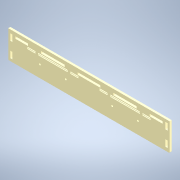
# Autodesk Inventor part: case bottom front
Saved by Autodesk Inventor 2022 (Build 260153000, 153)
## iProperties
Created: 2021-05-28
Part Number: case bottom front
Material: Nylon, molybdenum disulphide
Document SubType Name: Modeling
Designer: benka
Density: 1.13 g/cm^3
Appearance: Nylon 6
Author: benka
Autodesk Inventor part; units mm, degrees
ref_plane "YZ Plane" through (0, 0, 0) normal (1, 0, 0) x (0, 1, 0)
ref_plane "XZ Plane" through (0, 0, 0) normal (0, 1, 0) x (-1, 0, 0)
ref_plane "XY Plane" through (0, 0, 0) normal (0, 0, 1) x (1, 0, 0)
sketch "Sketch1" plane through (0, 0, 0) normal (0, 0, 1) x (1, 0, 0)
  circle A0 centre (-5.8379, -1.3582) radius 2
  circle A1 centre (54.1621, -1.3582) radius 2
  line L0 (81.6621, 21.6418) -> (111.6621, 21.6418) projected
  line L1 (111.6621, 21.6418) -> (111.6621, 26.6418) projected
  line L2 (81.6621, 26.6418) -> (111.6621, 26.6418) projected
  line L3 (81.6621, 21.6418) -> (81.6621, 26.6418) projected
  line L4 (-3.3379, 21.6418) -> (51.6621, 21.6418) projected
  line L5 (51.6621, 21.6418) -> (51.6621, 26.6418) projected
  line L6 (-3.3379, 26.6418) -> (51.6621, 26.6418) projected
  line L7 (-3.3379, 21.6418) -> (-3.3379, 26.6418) projected
  line L8 (-86.3379, 21.6418) -> (-33.3379, 21.6418) projected
  line L9 (-33.3379, 21.6418) -> (-33.3379, 26.6418) projected
  line L10 (-86.3379, 26.6418) -> (-33.3379, 26.6418) projected
  line L11 (-86.3379, 21.6418) -> (-86.3379, 26.6418) projected
  line L12 (-171.3379, 21.6418) -> (-116.3379, 21.6418) projected
  line L13 (-116.3379, 21.6418) -> (-116.3379, 26.6418) projected
  line L14 (-171.3379, 26.6418) -> (-116.3379, 26.6418) projected
  line L15 (-171.3379, 21.6418) -> (-171.3379, 26.6418) projected
  line L16 (-231.3379, 21.6418) -> (-201.3379, 21.6418) projected
  line L17 (-201.3379, 21.6418) -> (-201.3379, 26.6418) projected
  line L18 (-231.3379, 26.6418) -> (-201.3379, 26.6418) projected
  line L19 (-231.3379, 21.6418) -> (-231.3379, 26.6418) projected
  line L20 (126.1621, -31.3589) -> (-245.8379, -31.3589)
  line L21 (-247.8379, -29.3589) -> (-247.8379, 34.6418)
  line L22 (128.1621, -29.3589) -> (128.1621, 34.6418)
  line L23 (-247.8379, 34.6418) -> (128.1621, 34.6418)
  arc A2 (-247.8379, -29.3589) -> (-245.8379, -31.3589) centre (-245.8379, -29.3589) ccw
  arc A3 (126.1621, -31.3589) -> (128.1621, -29.3589) centre (126.1621, -29.3589) ccw
  line L24 (123.1621, -23.3589) -> (123.1621, -8.3597) projected
  line L25 (123.1621, -8.3597) -> (118.1621, -8.3597) projected
  line L26 (118.1621, -23.3589) -> (118.1621, -8.3597) projected
  line L27 (123.1621, -23.3589) -> (118.1621, -23.3589) projected
  line L28 (123.1621, 11.6403) -> (123.1621, 26.6418) projected
  line L29 (123.1621, 26.6418) -> (118.1621, 26.6418) projected
  line L30 (118.1621, 11.6403) -> (118.1621, 26.6418) projected
  line L31 (123.1621, 11.6403) -> (118.1621, 11.6403) projected
  line L32 (-237.8379, -23.3589) -> (-237.8379, -8.3597) projected
  line L33 (-237.8379, -8.3597) -> (-242.8379, -8.3597) projected
  line L34 (-242.8379, -23.3589) -> (-242.8379, -8.3597) projected
  line L35 (-237.8379, -23.3589) -> (-242.8379, -23.3589) projected
  line L36 (-237.8379, 11.6403) -> (-237.8379, 26.6418) projected
  line L37 (-237.8379, 26.6418) -> (-242.8379, 26.6418) projected
  line L38 (-242.8379, 11.6403) -> (-242.8379, 26.6418) projected
  line L39 (-237.8379, 11.6403) -> (-242.8379, 11.6403) projected
  line L40 (-201.8409, 14.8575) -> (-185.8409, 14.8575)
  line L41 (-185.8409, 19.8575) -> (-201.8409, 19.8575)
  line L42 (-85.8409, 14.8575) -> (-101.8409, 14.8575)
  line L43 (-101.8409, 19.8575) -> (-85.8409, 19.8575)
  line L44 (-176.8409, 14.8575) -> (-110.8409, 14.8575)
  line L45 (-110.8409, 19.8575) -> (-176.8409, 19.8575)
  arc A4 (-178.8409, 16.8575) -> (-176.8409, 14.8575) centre (-176.8409, 16.8575) ccw
  arc A5 (-108.8409, 17.8575) -> (-110.8409, 19.8575) centre (-110.8409, 17.8575) ccw
  arc A6 (-110.8409, 14.8575) -> (-108.8409, 16.8575) centre (-110.8409, 16.8575) ccw
  arc A7 (-103.8409, 16.8575) -> (-101.8409, 14.8575) centre (-101.8409, 16.8575) ccw
  arc A8 (-101.8409, 19.8575) -> (-103.8409, 17.8575) centre (-101.8409, 17.8575) ccw
  arc A9 (-83.8409, 17.8575) -> (-85.8409, 19.8575) centre (-85.8409, 17.8575) ccw
  arc A10 (-85.8409, 14.8575) -> (-83.8409, 16.8575) centre (-85.8409, 16.8575) ccw
  arc A11 (-183.8409, 17.8575) -> (-185.8409, 19.8575) centre (-185.8409, 17.8575) ccw
  arc A12 (-185.8409, 14.8575) -> (-183.8409, 16.8575) centre (-185.8409, 16.8575) ccw
  arc A13 (-203.8409, 16.8575) -> (-201.8409, 14.8575) centre (-201.8409, 16.8575) ccw
  arc A14 (-201.8409, 19.8575) -> (-203.8409, 17.8575) centre (-201.8409, 17.8575) ccw
  arc A15 (-176.8409, 19.8575) -> (-178.8409, 17.8575) centre (-176.8409, 17.8575) ccw
  line L46 (-203.8409, 16.8575) -> (-183.8409, 16.8575)
  line L47 (-183.8409, 17.8575) -> (-203.8409, 17.8575)
  line L48 (-178.8409, 16.8575) -> (-108.8409, 16.8575)
  line L49 (-108.8409, 17.8575) -> (-178.8409, 17.8575)
  line L50 (-103.8409, 16.8575) -> (-83.8409, 16.8575)
  line L51 (-83.8409, 17.8575) -> (-103.8409, 17.8575)
  line L52 (57.1591, 19.8575) -> (-8.8409, 19.8575)
  line L53 (-8.8409, 14.8575) -> (57.1591, 14.8575)
  line L54 (59.1591, 17.8575) -> (-10.8409, 17.8575)
  line L55 (-10.8409, 16.8575) -> (59.1591, 16.8575)
  arc A16 (59.1591, 17.8575) -> (57.1591, 19.8575) centre (57.1591, 17.8575) ccw
  arc A17 (57.1591, 14.8575) -> (59.1591, 16.8575) centre (57.1591, 16.8575) ccw
  arc A18 (64.1591, 16.8575) -> (66.1591, 14.8575) centre (66.1591, 16.8575) ccw
  arc A19 (66.1591, 19.8575) -> (64.1591, 17.8575) centre (66.1591, 17.8575) ccw
  line L56 (82.1591, 14.8575) -> (66.1591, 14.8575)
  line L57 (66.1591, 19.8575) -> (82.1591, 19.8575)
  arc A20 (82.1591, 14.8575) -> (84.1591, 16.8575) centre (82.1591, 16.8575) ccw
  arc A21 (84.1591, 17.8575) -> (82.1591, 19.8575) centre (82.1591, 17.8575) ccw
  line L58 (-33.8409, 14.8575) -> (-17.8409, 14.8575)
  line L59 (-17.8409, 19.8575) -> (-33.8409, 19.8575)
  arc A22 (-10.8409, 16.8575) -> (-8.8409, 14.8575) centre (-8.8409, 16.8575) ccw
  arc A23 (-8.8409, 19.8575) -> (-10.8409, 17.8575) centre (-8.8409, 17.8575) ccw
  arc A24 (-17.8409, 14.8575) -> (-15.8409, 16.8575) centre (-17.8409, 16.8575) ccw
  arc A25 (-15.8409, 17.8575) -> (-17.8409, 19.8575) centre (-17.8409, 17.8575) ccw
  arc A26 (-33.8409, 19.8575) -> (-35.8409, 17.8575) centre (-33.8409, 17.8575) ccw
  line L60 (-35.8409, 16.8575) -> (-15.8409, 16.8575)
  line L61 (-15.8409, 17.8575) -> (-35.8409, 17.8575)
  arc A27 (-35.8409, 16.8575) -> (-33.8409, 14.8575) centre (-33.8409, 16.8575) ccw
  line L62 (64.1591, 16.8575) -> (84.1591, 16.8575)
  line L63 (84.1591, 17.8575) -> (64.1591, 17.8575)
  circle A28 centre (-173.8379, -1.3582) radius 2
  circle A29 centre (-113.8379, -1.3582) radius 2
  line L64 (-237.8379, -31.3589) -> (-242.8379, -31.3589) projected
  point P0 (24.1621, -1.3582)
  point P1 (-203.8409, 14.8575)
  point P2 (-203.8409, 19.8575)
  point P3 (-35.8409, 14.8575)
  point P4 (-35.8409, 19.8575)
  point P5 (-143.8379, -1.3582)
  dimension "d36" = 4
  dimension "d37" = 4
  dimension "d40" = 30
  dimension "d41" = 30
  dimension "d48" = 2
  dimension "d53" = 2
  dimension "d55" = 8
  dimension "d56" = 5
  dimension "d57" = 2
  dimension "d58" = 5
  dimension "d59" = 2
  dimension "d60" = 376
  dimension "d63" = 28
  dimension "d64" = 28
  dimension "d65" = 28
  dimension "d66" = 4
  dimension "d67" = 4
  dimension "d68" = 30
  dimension "d69" = 30
  dimension "d70" = 74
  dimension "d71" = 74
  dimension "d72" = 28
  dimension "d73" = 28
  dimension "d74" = 2.5
  dimension "d75" = 2.5
  dimension "d76" = 2.5
  dimension "d77" = 0
  constraints: 56 end point, 54 point on circle, 30 centre point, 16 point on line, 4 coincident, 4 tangent, 2 perpendicular, 1 horizontal, 1 vertical
  measures "d36" diameter of A0
  measures "d37" diameter of A1
  measures "d40" distance of point (54.162, -1.358) point (24.162, -1.358)
  measures "d41" distance of point (-5.838, -1.358) point (24.162, -1.358)
  measures "d48" radius of A2
  measures "d53" radius of A3
  measures "d55" distance between parallel lines of L23 L18
  measures "d56" distance of point (-203.841, 19.857) point (-203.841, 14.857)
  measures "d57" radius of A4
  measures "d58" distance of point (-35.841, 19.857) point (-35.841, 14.857)
  measures "d59" radius of A22
  measures "d60" distance between parallel lines of L22 L21
  measures "d63" distance from line of L10 A0.centre
  measures "d64" distance from line of L6 A1.centre
  measures "d65" distance from line of L6 point (24.162, -1.358)
  measures "d66" diameter of A28
  measures "d67" diameter of A29
  measures "d68" distance of point (-113.838, -1.358) point (-143.838, -1.358)
  measures "d69" distance of point (-173.838, -1.358) point (-143.838, -1.358)
  measures "d70" distance from line of L21 A28.centre
  measures "d71" distance from line of L22 A1.centre
  measures "d72" distance from line of L14 A29.centre
  measures "d73" distance from line of L14 point (-173.838, -1.358)
  measures "d74" horizontal distance of L6.start A0.centre
  measures "d75" horizontal distance of point (54.162, -1.358) L5.end
  measures "d76" horizontal distance of L14.start A28.centre
  measures "d77" distance between parallel lines of L20 L64
extrude "Extrusion1" add sketch "Sketch1" along normal blind 5
body "Solid1"
